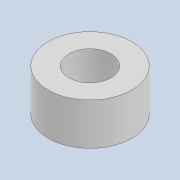
# Autodesk Inventor part: 垫圈
Saved by Autodesk Inventor 2020 (Build 240168000, 168)
## iProperties
Created: 2022-05-21
Part Number: 垫圈
Material: 常规
Document SubType Name: Modeling
Designer: 唐晨超
Density: 1 g/cm^3
Appearance: 默认
Author: 唐晨超
Autodesk Inventor part; units mm, degrees
ref_plane "YZ Plane" through (0, 0, 0) normal (1, 0, 0) x (0, 1, 0)
ref_plane "XZ Plane" through (0, 0, 0) normal (0, 1, 0) x (-1, 0, 0)
ref_plane "XY Plane" through (0, 0, 0) normal (0, 0, 1) x (1, 0, 0)
sketch "草图1" plane through (0, 0, 0) normal (0, 1, 0) x (-1, 0, 0)
  circle A0 centre (0, 0) radius 10
  circle A1 centre (0, 0) radius 5
  dimension "d0" = 20
  dimension "d3" = 10
  constraints: 2 centre point, 2 coincident
  measures "d0" diameter of A0
  measures "d3" diameter of A1
extrude "拉伸1" add sketch "草图1" along normal blind 10
equation "\"d0\" = d1"
equation "\"d3\" = d2"
equation "\"d4\" = h1"
equation "\"d1\" = 20"
equation "\"d2\" = 10"
equation "\"h1\" = 10"
